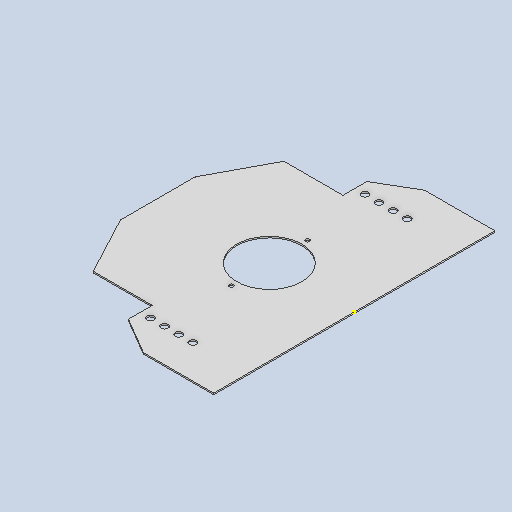
# Autodesk Inventor part: Peça3
Saved by Autodesk Inventor 2023 (Build 270158000, 158)
## iProperties
Created: 2023-08-07
Part Number: Peça3
Material: Genérico
Document SubType Name: Modeling
Designer: azeve
Density: 1 g/cm^3
Appearance: Padrão
Author: azeve
Autodesk Inventor part; units mm, degrees
ref_plane "YZ Plane" through (0, 0, 0) normal (1, 0, 0) x (0, 1, 0)
ref_plane "XZ Plane" through (0, 0, 0) normal (0, 1, 0) x (-1, 0, 0)
ref_plane "XY Plane" through (0, 0, 0) normal (0, 0, 1) x (1, 0, 0)
sketch "Esboço1" plane through (0, 0, 0) normal (0, 1, 0) x (-1, 0, 0)
  line L0 (0, 100) -> (50, 100)
  line L1 (50, 100) -> (75.8622, 84.7964)
  line L2 (50, 100) -> (80, 100) construction
  line L3 (75.8622, 84.7964) -> (75.8622, 67.7964)
  line L4 (75.8622, 67.7964) -> (117.8622, 67.7964)
  line L5 (117.8622, 67.7964) -> (170.8622, 67.7964) construction
  circle A0 centre (68.629, 76.2964) radius 2.5
  circle A1 centre (58.629, 76.2964) radius 2.5
  circle A2 centre (48.629, 76.2964) radius 2.5
  circle A3 centre (38.629, 76.2964) radius 2.5
  line L6 (0, -100) -> (50, -100)
  line L7 (50, -100) -> (75.8622, -84.7964)
  line L8 (75.8622, -84.7964) -> (75.8622, -67.7964)
  line L9 (75.8622, -67.7964) -> (117.8622, -67.7964)
  circle A4 centre (68.629, -76.2964) radius 2.5
  circle A5 centre (58.629, -76.2964) radius 2.5
  circle A6 centre (48.629, -76.2964) radius 2.5
  circle A7 centre (38.629, -76.2964) radius 2.5
  line L10 (0, 100) -> (0, -100)
  line L11 (75.8622, -82.1665) -> (75.8622, -70.1665)
  circle A8 centre (61.129, 0) radius 23
  line L12 (117.8622, 67.7964) -> (139.8134, 26.55)
  line L13 (117.8622, -67.7964) -> (139.8134, -26.55)
  line L14 (139.8134, 26.55) -> (139.8134, -26.55)
  line L15 (0, 0) -> (61.129, 0)
  circle A9 centre (59.9305, 27.5032) radius 1.5
  circle A10 centre (60.6516, -27.5032) radius 1.5
  dimension "d5" = 30
  dimension "d6" = 30.45
  dimension "d17" = 10
  dimension "d32" = 42
  dimension "d33" = 25.8621
  dimension "d34" = 50
  dimension "d37" = 46
  dimension "d40" = 53.1001
  dimension "d41" = 21.9513
  dimension "d42" = 17
  dimension "d43" = 46.7239
  dimension "d44" = 118.022
  dimension "d45" = 61.129
  dimension "d46" = 200
  dimension "d48" = 3
  dimension "d53" = 3
  constraints: 32 end point, 11 centre point, 5 horizontal, 3 vertical, 1 equal length, 1 perpendicular, 1 point on line, 6 other
  measures "d5" distance of L0.end L1.end
  measures "d6" angle of L1 L2
  measures "d17" distance of A0.centre A1.centre
  measures "d32" distance of L8.end L9.end
  measures "d33" horizontal distance of L7.end L6.end
  measures "d34" distance of L6.start L6.end
  measures "d37" diameter of A8
  measures "d40" distance of L12.end L13.end
  measures "d41" horizontal distance of L9.end L13.end
  measures "d42" distance of L1.end L3.end
  measures "d43" distance of L4.end L12.end
  measures "d44" angle of L12 L4
  measures "d45" distance of L15.start L15.end
  measures "d46" distance of L0.start L6.start
  measures "d48" diameter of A9
  measures "d53" diameter of A10
extrude "Extrusão1" add sketch "Esboço1" along normal blind 1 contours A8 | L0 L1 L3 L4 L12 L14 L13 L9 L8 L7 L6 L10 | A9 | A10
sketch "Esboço3" plane through (0, 1, 0) normal (0, 1, 0) x (1, 0, 0)
  circle A0 centre (-60.4361, 0) radius 23.1709
  point P0 (0, 0)
  constraints: 1 centre point
extrude "Extrusão3" cut sketch "Esboço3" against normal blind 3.75
extrude "Extrusão4" cut sketch "Esboço1" along normal blind 3.75 contours A9
extrude "Extrusão5" [suppressed]
extrude "Extrusão6" cut sketch "Esboço1" along normal blind 3.75 contours A10
sketch "Esboço4" plane through (0, 1, 0) normal (0, 1, 0) x (1, 0, 0)
  point P0 (0, 0)
